Autodesk Inventor part; units mm, degrees
(part 2 of 2)
  arc A219 (-10.9587, 27.3479) -> (-10.6477, 23.9348) centre (-8.0778, 25.8897) ccw
  arc A220 (-8.54, 24.7486) -> (-10.5209, 27.4724) centre (-11.5467, 24.6442) ccw
  line L86 (-14.0887, 25.825) -> (-14.5061, 25.6432)
  arc A221 (-14.5061, 25.6432) -> (-13.7429, 22.302) centre (-11.4565, 24.582) ccw
  arc A222 (-11.7625, 23.3895) -> (-14.0887, 25.825) centre (-14.7284, 22.8853) ccw
  line L87 (-17.4052, 23.7167) -> (-17.7946, 23.4809)
  arc A223 (-17.7946, 23.4809) -> (-16.5929, 20.2713) centre (-14.6307, 22.8357) ccw
  arc A224 (-14.775, 21.613) -> (-17.4052, 23.7167) centre (-17.6473, 20.718) ccw
  line L88 (-20.411, 21.1852) -> (-20.7655, 20.8996)
  arc A225 (-20.7655, 20.8996) -> (-19.1467, 17.8788) centre (-17.5439, 20.6819) ccw
  arc A226 (-17.5239, 19.4508) -> (-20.411, 21.1852) centre (-20.2513, 18.181) ccw
  line L89 (-23.0526, 18.2757) -> (-23.3659, 17.9454)
  arc A227 (-23.3659, 17.9454) -> (-21.3589, 15.1673) centre (-20.144, 18.159) ccw
  arc A228 (-19.9601, 16.9416) -> (-23.0526, 18.2757) centre (-22.4939, 15.3195) ccw
  line L90 (-25.2828, 15.04) -> (-25.5493, 14.6709)
  arc A229 (-25.5493, 14.6709) -> (-23.1899, 12.1851) centre (-22.3846, 15.312) ccw
  arc A230 (-22.0401, 14.13) -> (-25.2828, 15.04) centre (-24.3351, 12.1847) ccw
  line L91 (-27.0619, 11.5359) -> (-27.2767, 11.1346)
  arc A231 (-27.2767, 11.1346) -> (-24.6071, 8.9854) centre (-24.2257, 12.1918) ccw
  arc A232 (-23.7268, 11.0662) -> (-27.0619, 11.5359) centre (-25.742, 8.8324) ccw
  line L92 (-28.358, 7.826) -> (-28.5175, 7.3996)
  arc A233 (-28.5175, 7.3996) -> (-25.5852, 5.6255) centre (-25.6346, 8.854) ccw
  arc A234 (-24.9901, 7.805) -> (-28.358, 7.826) centre (-26.6896, 5.3225) ccw
  line L93 (-29.1481, 3.9764) -> (-29.2493, 3.5326)
  arc A235 (-29.2493, 3.5326) -> (-26.1067, 2.1651) centre (-26.586, 5.3583) ccw
  arc A236 (-25.8074, 4.4045) -> (-29.1481, 3.9764) centre (-27.1609, 1.7177) ccw
  arc A237 (-24.989, -8.2622) -> (-24.5929, -9.3755) centre (0, 0) ccw
  arc A238 (-23.6648, -11.5192) -> (-23.1239, -12.5698) centre (0, 0) ccw
  arc A239 (-21.9183, -14.5706) -> (-21.2422, -15.5397) centre (0, 0) ccw
  arc A240 (-19.7806, -17.362) -> (-18.9814, -18.2324) centre (0, 0) ccw
  arc A241 (-17.29, -19.8436) -> (-16.3819, -20.5997) centre (0, 0) ccw
  arc A242 (-14.4908, -21.9711) -> (-13.4901, -22.5993) centre (0, 0) ccw
  arc A243 (-11.4331, -23.7065) -> (-10.3575, -24.1958) centre (0, 0) ccw
  arc A244 (-8.1713, -25.0188) -> (-7.0401, -25.3604) centre (0, 0) ccw
  arc A245 (-4.7637, -25.8847) -> (-3.5971, -26.0725) centre (0, 0) ccw
  arc A246 (-1.2711, -26.2887) -> (-0.0899, -26.3193) centre (0, 0) ccw
  arc A247 (2.2442, -26.2236) -> (3.4189, -26.0964) centre (0, 0) ccw
  arc A248 (5.7194, -25.6905) -> (6.8668, -25.4079) centre (0, 0) ccw
  arc A249 (9.0926, -24.6989) -> (10.192, -24.2659) centre (0, 0) ccw
  arc A250 (12.3035, -23.2666) -> (13.3354, -22.6909) centre (0, 0) ccw
  arc A251 (15.2949, -21.4191) -> (16.2408, -20.711) centre (0, 0) ccw
  arc A252 (18.0133, -19.1894) -> (18.8564, -18.3616) centre (0, 0) ccw
  arc A253 (20.4103, -16.6173) -> (21.1356, -15.6844) centre (0, 0) ccw
  arc A254 (22.443, -13.7486) -> (23.0375, -12.7274) centre (0, 0) ccw
  arc A255 (24.0753, -10.6346) -> (24.5283, -9.5432) centre (0, 0) ccw
  arc A256 (25.2779, -7.3307) -> (25.5815, -6.1888) centre (0, 0) ccw
  arc A257 (26.0295, -3.8961) -> (26.1781, -2.7239) centre (0, 0) ccw
  arc A258 (26.3165, -0.392) -> (26.3076, 0.7896) centre (0, 0) ccw
  arc A259 (26.1339, 3.1192) -> (25.9676, 4.289) centre (0, 0) ccw
  arc A260 (25.485, 6.5747) -> (25.1642, 7.7119) centre (0, 0) ccw
  arc A261 (24.3813, 9.9128) -> (23.9118, 10.9972) centre (0, 0) ccw
  arc A262 (22.8425, 13.0741) -> (22.2327, 14.0862) centre (0, 0) ccw
  arc A263 (20.8961, 16.002) -> (20.1568, 16.9238) centre (0, 0) ccw
  arc A264 (18.5768, 18.6444) -> (17.7212, 19.4595) centre (0, 0) ccw
  arc A265 (15.926, 20.9541) -> (14.9694, 21.6478) centre (0, 0) ccw
  arc A266 (12.991, 22.8899) -> (11.9505, 23.4499) centre (0, 0) ccw
  arc A267 (9.8241, 24.4172) -> (8.7183, 24.8335) centre (0, 0) ccw
  arc A268 (6.482, 25.5087) -> (5.3305, 25.774) centre (0, 0) ccw
  arc A269 (3.0242, 26.1451) -> (1.8476, 26.2545) centre (0, 0) ccw
  arc A270 (-0.4876, 26.3149) -> (-1.6683, 26.2665) centre (0, 0) ccw
  arc A271 (-3.9907, 26.0151) -> (-5.1544, 25.8098) centre (0, 0) ccw
  arc A272 (-7.4226, 25.2511) -> (-8.5485, 24.8925) centre (0, 0) ccw
  arc A273 (-10.722, 24.0365) -> (-11.79, 23.531) centre (0, 0) ccw
  arc A274 (-13.8301, 22.3929) -> (-14.8212, 21.7496) centre (0, 0) ccw
  arc A275 (-16.6913, 20.3497) -> (-17.5879, 19.58) centre (0, 0) ccw
  arc A276 (-19.2548, 17.9434) -> (-20.0407, 17.0611) centre (0, 0) ccw
  arc A277 (-21.4746, 15.2169) -> (-22.136, 14.2377) centre (0, 0) ccw
  arc A278 (-23.3112, 12.2189) -> (-23.8361, 11.1602) centre (0, 0) ccw
  arc A279 (-24.7318, 9.0028) -> (-25.111, 7.8836) centre (0, 0) ccw
  arc A280 (-25.7111, 5.626) -> (-25.9377, 4.4663) centre (0, 0) ccw
  arc A281 (-26.2316, 2.1488) -> (-26.3016, 0.9693) centre (0, 0) ccw
  arc A282 (-26.2839, -1.3667) -> (-26.1961, -2.545) centre (0, 0) ccw
  arc A283 (-25.8672, -4.8578) -> (-25.6231, -6.0139) centre (0, 0) ccw
  line L94 (1.3564, 15.5941) -> (5.7598, 19.9975) construction
  line L95 (5.763, 20.0007) -> (-5.4898, 23.9965)
  line L96 (0.1396, 24.9441) -> (0.0163, 24.8855)
  line L97 (-7.5731, 21.9421) -> (-3.7017, 10.536)
  arc A284 (-3.7017, 10.536) -> (5.763, 20.0007) centre (1.0307, 15.2684) ccw
  arc A285 (-5.4898, 23.9965) -> (-7.5731, 21.9421) centre (-6.0338, 22.4646) ccw
  line L98 (-22.789, 4.4125) -> (-10.9753, 2.0623)
  arc A286 (-10.9753, 2.0623) -> (-14.4396, 14.9913) centre (-12.7074, 8.5268) ccw
  line L99 (-12.8267, 8.9717) -> (-14.4384, 14.9869) construction
  arc A287 (-23.5265, 7.2439) -> (-22.789, 4.4125) centre (-22.4718, 6.0069) ccw
  line L100 (-14.4396, 14.9913) -> (-23.5265, 7.2439)
  line L101 (-15.2159, -17.5296) -> (-7.2736, -8.4737)
  arc A288 (-7.2736, -8.4737) -> (-20.2026, -5.0094) centre (-13.7381, -6.7416) ccw
  line L102 (-14.183, -6.6224) -> (-20.1982, -5.0106) construction
  arc A289 (-18.0367, -16.7526) -> (-15.2159, -17.5296) centre (-16.438, -16.4577) ccw
  line L103 (-20.2026, -5.0094) -> (-18.0367, -16.7526)
  line L104 (7.5731, -21.9421) -> (3.7017, -10.536)
  arc A290 (3.7017, -10.536) -> (-5.763, -20.0007) centre (-1.0307, -15.2684) ccw
  line L105 (-1.3564, -15.5941) -> (-5.7598, -19.9975) construction
  arc A291 (5.4898, -23.9965) -> (7.5731, -21.9421) centre (6.0338, -22.4646) ccw
  line L106 (-5.763, -20.0007) -> (5.4898, -23.9965)
  line L107 (22.789, -4.4125) -> (10.9753, -2.0623)
  arc A292 (10.9753, -2.0623) -> (14.4396, -14.9913) centre (12.7074, -8.5268) ccw
  line L108 (12.8267, -8.9717) -> (14.4384, -14.9869) construction
  arc A293 (23.5265, -7.2439) -> (22.789, -4.4125) centre (22.4718, -6.0069) ccw
  line L109 (14.4396, -14.9913) -> (23.5265, -7.2439)
  line L110 (15.2159, 17.5296) -> (7.2736, 8.4737)
  arc A294 (7.2736, 8.4737) -> (20.2026, 5.0094) centre (13.7381, 6.7416) ccw
  line L111 (14.183, 6.6224) -> (20.1982, 5.0106) construction
  arc A295 (18.0367, 16.7526) -> (15.2159, 17.5296) centre (16.438, 16.4577) ccw
  line L112 (20.2026, 5.0094) -> (18.0367, 16.7526)
  point P0 (2.7665, -46.0619)
  point P1 (-2.7665, -46.0619)
  dimension "d95" = 360
  dimension "d96" = 1.6256
  dimension "d97" = 360
  constraints: 306 point on circle, 132 end point, 107 centre point, 2 tangent, 645 other
  measures "d96" radius of A285
extrude "Extrusion17" add sketch "Sketch20" against normal blind 5.715 contours A192 A258 A189 A141 A140 A139 A190 A257 A187 A138 A137 A136 A188 A256 A185 A135 A134 A133 A186 A255 A183 A132 A131 A130 A184 A254 A181 A129 A128 A127 A182 A253 A179 A126 A125 A124 A180 A252 A177 A123 A122 A121 A178 A251 A175 A120 A119 A118 A176 A250 A173 A117 A116 A115 A174 A249 A171 A114 A113 A112 A172 A248 A169 A111 A110 A109 A170 A247 A167 A108 A107 A106 A168 A246 A165 A105 A104 A103 A166 A245 A163 A102 A101 A100 A164 A244 A161 A99 A98 A97 A162 A243 A159 A96 A95 A94 A160 A242 A157 A93 A92 A91 A158 A241 A155 A90 A89 A88 A156 A240 A153 A87 A86 A85 A154 A239 A151 A84 A83 A82 A152 A238 A149 A81 A80 A79 A150 A237 A147 A78 A77 A76 A148 A283 A145 A75 A74 A73 A146 A282 A143 A72 A71 A70 A144 A281 A235 A69 A68 A67 A236 A280 A233 A66 A65 A64 A234 A279 A231 A63 A62 A61 A232 A278 A229 A60 A59 A58 A230 A277 A227 A57 A56 A55 A228 A276 A225 A54 A53 A52 A226 A275 A223 A51 A50 A49 A224 A274 A221 A48 A47 A46 A222 A273 A219 A45 A44 A43 A220 A272 A217 A42 A41 A40 A218 A271 A215 A39 A38 A37 A216 A270 A213 A36 A35 A34 A214 A269 A211 A33 A32 A31 A212 A268 A209 A30 A29 A28 A210 A267 A207 A27 A26 A25 A208 A266 A205 A24 A23 A22 A206 A265 A203 A21 A20 A19 A204 A264 A201 A18 A17 A16 A202 A263 A199 A15 A14 A13 A200 A262 A197 A12 A11 A10 A198 A261 A195 A9 A8 A7 A196 A260 A193 A6 A5 A4 A194 A259 A191 A3 A2 A1 | A1 A2 A3 A191 L71 A192 | A189 L70 A190 A139 A140 A141 | A4 A5 A6 A193 L72 A194 | A187 L69 A188 A136 A137 A138 | A7 A8 A9 A195 L73 A196 | A185 L68 A186 A133 A134 A135 | A10 A11 A12 A197 L74 A198 | A183 L67 A184 A130 A131 A132 | A13 A14 A15 A199 L75 A200 | A181 L66 A182 A127 A128 A129 | A16 A17 A18 A201 L76 A202 | A179 L65 A180 A124 A125 A126 | A19 A20 A21 A203 L77 A204 | A177 L64 A178 A121 A122 A123 | A22 A23 A24 A205 L78 A206 | A175 L63 A176 A118 A119 A120 | A25 A26 A27 A207 L79 A208 | A173 L62 A174 A115 A116 A117 | A28 A29 A30 A209 L80 A210 | A171 L61 A172 A112 A113 A114 | A31 A32 A33 A211 L81 A212 | A169 L60 A170 A109 A110 A111 | A34 A35 A36 A213 L82 A214 | A167 L59 A168 A106 A107 A108 | A37 A38 A39 A215 L83 A216 | A165 L58 A166 A103 A104 A105 | A40 A41 A42 A217 L84 A218 | A163 L57 A164 A100 A101 A102 | A43 A44 A45 A219 L85 A220 | A161 L56 A162 A97 A98 A99 | A46 A47 A48 A221 L86 A222 | A159 L55 A160 A94 A95 A96 | A49 A50 A51 A223 L87 A224 | A157 L54 A158 A91 A92 A93 | A52 A53 A54 A225 L88 A226 | A155 L53 A156 A88 A89 A90 | A55 A56 A57 A227 L89 A228 | A153 L52 A154 A85 A86 A87 | A58 A59 A60 A229 L90 A230 | A151 L51 A152 A82 A83 A84 | A61 A62 A63 A231 L91 A232 | A149 L50 A150 A79 A80 A81 | A64 A65 A66 A233 L92 A234 | A147 L49 A148 A76 A77 A78 | A67 A68 A69 A235 L93 A236 | A145 L48 A146 A73 A74 A75 | A70 A71 A72 A143 L47 A144
sketch "Sketch21" plane through (2.7665, 46.0619, 14.665) normal (0, 0, -1) x (-1, 0, 0)
  circle A0 centre (0, 0) radius 7.5 projected
  arc A1 (-26.2839, -1.3667) -> (-26.1961, -2.545) centre (0, 0) ccw projected
  circle A2 centre (0, 0) radius 7.5
  point P0 (2.7665, -46.0619)
  dimension "d114" = 15
  constraints: 1 centre point, 1 coincident, 1 concentric
  measures "d114" diameter of A0
extrude "Extrusion19" add sketch "Sketch21" against normal up to next
sketch "Sketch22" plane through (2.7665, 46.0619, 14.665) normal (0, 0, -1) x (-1, 0, 0)
  arc A0 (-26.2839, -1.3667) -> (-26.1961, -2.545) centre (0, 0) ccw projected
  circle A1 centre (0, 0) radius 7.5057
  point P0 (2.7665, -46.0619)
  dimension "d115" = 15.0114
  constraints: 1 centre point, 1 coincident
  measures "d115" diameter of A1
extrude "Extrusion20" add sketch "Sketch22" along normal blind 4.6
sketch "Sketch23" plane through (2.7665, 46.0619, 30.968) normal (0, 0, 1) x (1, 0, 0)
  arc A0 (2.5663, 39.2863) -> (0.9579, 39.3583) centre (0, 0) ccw projected
  line L0 (0, -4.792) -> (-4.15, -2.396)
  line L1 (-4.15, -2.396) -> (-4.15, 2.396)
  line L2 (-4.15, 2.396) -> (0, 4.792)
  line L3 (0, 4.792) -> (4.15, 2.396)
  line L4 (4.15, 2.396) -> (4.15, -2.396)
  line L5 (4.15, -2.396) -> (0, -4.792)
  point P0 (-2.7665, -46.0619)
  dimension "d118" = 8.3
  constraints: 12 end point, 1 coincident, 13 other
  measures "d118" distance between parallel lines of L4 L1
extrude "Extrusion21" cut sketch "Sketch23" against normal blind 4
sketch "Sketch24" plane through (2.7665, 46.0619, 10.065) normal (0, 0, -1) x (-1, 0, 0)
  circle A0 centre (0, 0) radius 7.5057 projected
  circle A1 centre (0, 0) radius 2.65
  point P0 (2.7665, -46.0619)
  dimension "d121" = 5.3
  constraints: 1 centre point, 1 coincident
  measures "d121" diameter of A1
extrude "Extrusion22" cut sketch "Sketch24" against normal through all contours A1
sketch "Sketch25" plane through (2.7665, 46.0619, 10.065) normal (0, 0, -1) x (-1, 0, 0)
  circle A0 centre (0, 0) radius 2.65 projected
  circle A1 centre (0, 0) radius 7.5057 projected
  circle A2 centre (0, 0) radius 4
  point P0 (2.7665, -46.0619)
  dimension "d124" = 8
  constraints: 1 centre point, 1 coincident
  measures "d124" diameter of A2
extrude "Extrusion23" add sketch "Sketch25" along normal blind 6 contours A2
body "Solid1"
